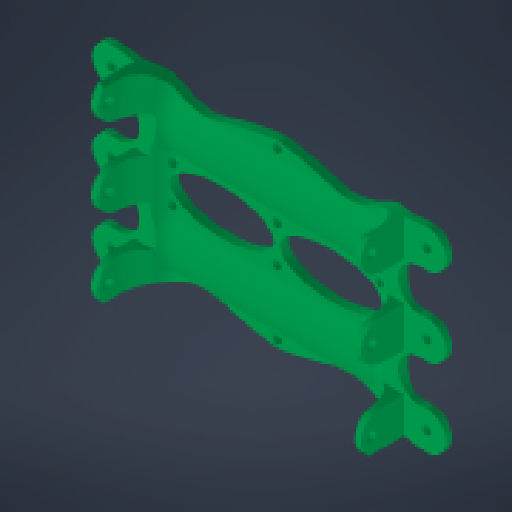
# Autodesk Inventor part: motor_holder_down
Saved by Autodesk Inventor 2024 (Build 280153000, 153)
## iProperties
Created: 2023-09-25
Part Number: motor_holder_down
Material: Типовые
Document SubType Name: Modeling
Designer: user
Mass: 66.3399 g
Surface Area: 381.903 cm^2
Volume: 66.3399 cm^3
Density: 1 g/cm^3
Appearance: По умолчанию
Author: user
Autodesk Inventor part; units mm, degrees
ref_plane "YZ Plane" through (0, 0, 0) normal (1, 0, 0) x (0, 1, 0)
sketch "Эскиз1" plane through (0, 0, 0) normal (0, 0, 1) x (1, 0, 0)
  line L0 (0, 0) -> (0, 20)
  line L1 (0, 20) -> (-20, 20)
  line L2 (-20, 20) -> (-20, 23)
  line L3 (-20, 23) -> (0, 23)
  line L4 (10, 27.5) -> (60, 27.5)
  line L5 (60, 27.5) -> (60, 23.5)
  line L6 (3, 23.5) -> (60, 23.5)
  line L7 (0, 23) -> (10, 27.5)
  line L8 (3, 23.5) -> (3, 0)
  line L9 (3, 0) -> (0, 0)
  dimension "d1" = 20
  dimension "d2" = 20
  dimension "d5" = 3
  dimension "d41" = 4
  dimension "d42" = 60
  dimension "d43" = 50
  dimension "d45" = 3
  dimension "d46" = 23.5
  constraints: 20 end point, 5 perpendicular, 3 horizontal, 1 vertical, 1 vertical alignment
  measures "d1" distance of L0.end L1.end
  measures "d2" distance of L0.start L0.end
  measures "d5" distance of L1.end L2.end
  measures "d41" distance of L4.end L5.end
  measures "d42" horizontal distance of L3.end L4.end
  measures "d43" distance of L4.start L4.end
  measures "d45" distance of L8.end L0.start
  measures "d46" distance of L6.start L8.end
extrude "Выдавливание1" add sketch "Эскиз1" along normal blind 90
ref_plane "РабПлоскость1" through (0, 0, 45) normal (0, 0, 1) x (1, 0, 0)
sketch "Эскиз2" plane through (60, 23.5, 0) normal (1, 0, 0) x (0, 0, -1)
  line L0 (0, 4) -> (-90, 4) construction
  arc A0 (-32.8167, 4) -> (-11.1833, 4) centre (-22, 22) ccw
  line L1 (0, 4) -> (-90, 4) construction
  arc A1 (-11.1833, 4) -> (-32.8167, 4) centre (-22, 22) ccw construction
  arc A2 (-78.8167, 4) -> (-57.1833, 4) centre (-68, 22) ccw
  arc A3 (-57.1833, 4) -> (-78.8167, 4) centre (-68, 22) ccw construction
  line L2 (-68, 22) -> (-22, 22) construction
  line L3 (-11.1833, 4) -> (-32.8167, 4)
  line L4 (-57.1833, 4) -> (-78.8167, 4)
  point P0 (0, -23.5)
  point P1 (-45, 22)
  point P2 (-45, 4)
  point P3 (-57.1833, 4)
  dimension "d38" = 21
  dimension "d39" = 46
  dimension "d40" = 18
  constraints: 9 point on circle, 7 point on line, 6 end point, 4 centre point, 2 coincident, 2 concentric, 2 midpoint, 1 collinear, 1 equal radius, 1 horizontal, 1 horizontal alignment, 1 vertical alignment
  measures "d38" radius of A1
  measures "d39" distance of A0.centre A2.centre
  measures "d40" vertical distance of L0.end A2.centre
extrude "Выдавливание3" cut sketch "Эскиз2" against normal through all
sketch "Эскиз10" plane through (3, 0, 90) normal (1, 0, 0) x (0, 0, -1)
  circle A0 centre (10, 5.75) radius 2
  circle A1 centre (45, 5.75) radius 2
  circle A2 centre (80, 5.75) radius 2
  line L0 (0, 0) -> (0, 23.5) projected
  line L1 (10, 5.75) -> (45, 5.75) construction
  line L2 (45, 5.75) -> (80, 5.75) construction
  point P0 (90, 0)
  point P1 (0, 5.75)
  point P2 (0, 11.5)
  dimension "d48" = 4
  dimension "d49" = 10
  dimension "d50" = 10
  constraints: 4 end point, 3 centre point, 2 collinear, 2 equal radius, 2 horizontal alignment, 1 horizontal, 1 point on line
  measures "d48" diameter of A0
  measures "d49" horizontal distance of L0.start L1.start
  measures "d50" horizontal distance of point (90, 0) L2.end
extrude "Выдавливание8" cut sketch "Эскиз10" against normal through all
sketch "Эскиз11" plane through (-20, 23, 0) normal (0, 1, 0) x (1, 0, 0)
  circle A0 centre (10, -80) radius 2
  circle A1 centre (10, -45) radius 2
  circle A2 centre (10, -10) radius 2
  line L0 (20, -90) -> (0, -90) projected
  line L1 (20, 0) -> (0, 0) projected
  line L2 (10, -80) -> (10, -45) construction
  line L3 (10, -10) -> (10, -45) construction
  point P0 (10, -90)
  dimension "d53" = 10
  dimension "d54" = 10
  dimension "d55" = 4
  constraints: 4 end point, 3 centre point, 3 vertical alignment, 2 collinear, 2 equal radius, 1 midpoint, 1 vertical
  measures "d53" horizontal distance of L0.end L2.start
  measures "d54" distance from line of L1 L3.start
  measures "d55" diameter of A2
extrude "Выдавливание9" cut sketch "Эскиз11" against normal through all
fillet "Сопряжение2" radius 15 1 edges at (0, 23, 45)
sketch "Эскиз12" plane through (60, 23.5, 0) normal (1, 0, 0) x (0, 0, -1)
  line L0 (0, 0) -> (-90, 0) projected
  arc A0 (-78.8167, 0) -> (-57.1833, 0) centre (-68, 27.9821) ccw
  arc A1 (-32.8167, 0) -> (-11.1833, 0) centre (-22, 27.9821) ccw
  point P0 (-11.1833, 4)
  point P1 (-32.8167, 4)
  point P2 (-57.1833, 4)
  point P3 (-78.8167, 4)
  dimension "d60" = 30
  dimension "d61" = 30
  constraints: 4 point on circle, 4 point on line, 4 vertical alignment, 2 centre point
  measures "d60" radius of A0
  measures "d61" radius of A1
extrude "Выдавливание10" add sketch "Эскиз12" against normal up to surface (57 mm away)
fillet "Сопряжение3" radius 13 5 edges at (3, 21.4821, 68) (3, 21.4821, 22) (3, 23.5, 45) (3, 23.5, 5.5917) (3, 23.5, 84.4083)
mirror "Зеркальное отражение9" about plane through (60, 23.5, 0) normal (1, 0, 0) of "Выдавливание3", "Выдавливание8", "Выдавливание9", "Сопряжение2", "Выдавливание10", "Сопряжение3", "Выдавливание1"
sketch "Эскиз13" plane through (120, 0, 0) normal (1, 0, 0) x (0, 0, -1)
  line L0 (0, 20) -> (-90, 20) projected
  line L1 (0, 20) -> (-90, 20) projected
  line L2 (-54, 20) -> (-54, 10)
  line L3 (-36, 20) -> (-36, 10)
  arc A0 (-54, 10) -> (-36, 10) centre (-45, 10) ccw
  line L4 (-71, 20) -> (-71, 10)
  line L5 (-89, 20) -> (-89, 10)
  line L6 (-19, 20) -> (-19, 10)
  line L7 (-1, 20) -> (-1, 10)
  arc A1 (-89, 10) -> (-71, 10) centre (-80, 10) ccw
  arc A2 (-19, 10) -> (-1, 10) centre (-10, 10) ccw
  circle A3 centre (-80, 5.75) radius 2 projected
  circle A4 centre (-10, 5.75) radius 2 projected
  line L8 (-90, 20) -> (-90, 0) projected
  line L9 (0, 0) -> (-90, 0) projected
  line L10 (0, 20) -> (0, 0) projected
  point P0 (-45, 20)
  point P1 (-45, 20)
  dimension "d65" = 18
  dimension "d67" = 18
  dimension "d68" = 18
  dimension "d69" = 10
  constraints: 12 end point, 6 point on circle, 6 tangent, 5 vertical, 3 centre point, 3 vertical alignment, 1 horizontal alignment, 1 parallel, 1 perpendicular, 9 other
  measures "d65" distance between parallel lines of L3 L2
  measures "d67" distance between parallel lines of L5 L4
  measures "d68" distance of L7.start L6.start
  measures "d69" distance of L2.start L2.end
extrude "Выдавливание11" cut sketch "Эскиз13" against normal through all contours L10 L9 L8 L0 L5 A1 L4 L2 A0 L3 L6 A2 L7
sketch "Эскиз15" plane through (10, 27.5, 11.1833) normal (0, 1, 0) x (1, 0, 0)
  circle A0 centre (-20, 1.1833) radius 2 projected
  circle A1 centre (-20, -33.8167) radius 2 projected
  circle A2 centre (-20, -68.8167) radius 2 projected
  arc A3 (-19.2944, 9.654) -> (-18.446, -7.1734) centre (-20, 1.1833) ccw
  arc A4 (-18.446, -25.4599) -> (-18.446, -42.1734) centre (-20, -33.8167) ccw
  arc A5 (-18.446, -60.4599) -> (-19.2944, -77.2873) centre (-20, -68.8167) ccw
  arc A6 (-18.446, -25.4599) -> (-18.446, -7.1734) centre (-16.7458, -16.3167) ccw
  arc A7 (-18.446, -60.4599) -> (-18.446, -42.1734) centre (-16.7458, -51.3167) ccw
  line L0 (100, -67.6333) -> (0, -67.6333) projected
  line L1 (-30, 11.1833) -> (-30, -78.8167) projected
  line L2 (6, 11.1833) -> (94, 11.1833) projected
  line L3 (0, -78.8167) -> (100, -78.8167) projected
  line L4 (0, 11.1833) -> (100, 11.1833) projected
  line L5 (0, 11.1833) -> (-7.0641, 11.1833) projected
  line L6 (-7.0641, 11.1833) -> (-13.2195, 11.1833) projected
  line L7 (-13.2195, 11.1833) -> (-30, 11.1833) projected
  line L8 (-13.2195, -78.8167) -> (-30, -78.8167) projected
  line L9 (-13.2195, -78.8167) -> (-7.0641, -78.8167) projected
  line L10 (0, -78.8167) -> (-7.0641, -78.8167) projected
  arc A8 (7, 2.1833) -> (-19.2944, 9.654) centre (-25.1885, -61.1009) ccw
  arc A9 (-19.2944, -77.2873) -> (7, -69.8167) centre (-25.1885, -6.5324) ccw
  line L11 (7, 2.1833) -> (7, 11.1833)
  line L12 (7, -69.8167) -> (7, -78.8167)
  point P0 (-10, 11.1833)
  point P1 (-30, -33.8167)
  dimension "d72" = 17
  dimension "d73" = 9.3
  dimension "d79" = 9
  dimension "d80" = 37
  dimension "d81" = 71
  constraints: 14 point on circle, 7 centre point, 6 tangent, 4 end point, 3 coincident, 3 equal radius, 2 perpendicular, 2 point on line, 2 vertical alignment, 1 collinear, 1 midpoint
  measures "d72" diameter of A3
  measures "d73" radius of A7
  measures "d79" distance of L11.start L11.end
  measures "d80" distance of L1.start L11.end
  measures "d81" radius of A9
extrude "Выдавливание12" cut sketch "Эскиз15" against normal through all contours A3 A6 A4 A7 A5 A9 L12 L3 L10 L9 L8 L1 L7 L6 L5 L4 L2 L11 A8
ref_plane "РабПлоскость3" through (60, 10, 54) normal (-1, 0, 0) x (0, 0, 1)
mirror "Зеркальное отражение10" about plane through (60, 10, 54) normal (-1, 0, 0) of "Выдавливание12"
sketch "Эскиз16" plane through (10, 27.5, 57.1833) normal (0, 1, 0) x (1, 0, 0)
  arc A0 (7, 48.1833) -> (0, 51.2808) centre (-25.1885, -15.1009) ccw projected
  arc A1 (7, 48.1833) -> (26.0438, 46.6851) centre (18.334, 70.4665) ccw
  arc A2 (50, 52.1833) -> (26.0438, 46.6851) centre (69.2187, -86.4912) ccw
  line L0 (7, 57.1833) -> (93, 57.1833) projected
  line L1 (50, 52.1833) -> (50, 57.1833)
  line L2 (7, 57.1833) -> (7, 48.1833) projected
  point P0 (-10, 57.1833)
  dimension "d82" = 25
  dimension "d83" = 140
  dimension "d84" = 5
  constraints: 4 point on circle, 2 centre point, 2 end point, 2 tangent, 1 midpoint, 1 vertical, 1 vertical alignment
  measures "d82" radius of A1
  measures "d83" radius of A2
  measures "d84" distance of L1.start L1.end
extrude "Выдавливание13" cut sketch "Эскиз16" against normal through all
mirror "Зеркальное отражение11" about plane through (60, 10, 54) normal (-1, 0, 0) of "Выдавливание13"
mirror "Зеркальное отражение12" about plane through (0, 0, 45) normal (0, 0, 1) of "Выдавливание13", "Зеркальное отражение11"
sketch "Эскиз17" plane through (10, 27.5, 57.1833) normal (0, 1, 0) x (1, 0, 0)
  ellipse E0 centre (25.7195, 12.1833) end of major axis (48.7195, 12.1833) minor radius 10
  line L0 (113.2195, 3.2889) -> (113.2195, 21.0778) projected
  point P0 (-10, 57.1833)
  point P1 (113.2195, 12.1833)
  dimension "d88" = 23
  dimension "d89" = 10
  dimension "d90" = 87.5
  constraints: 1 centre point, 1 horizontal alignment, 1 midpoint, 1 other
  measures "d89" radius of E0
  measures "d90" distance of point (113.22, 12.183) E0.centre
extrude "Выдавливание14" cut sketch "Эскиз17" against normal through all
mirror "Зеркальное отражение13" about plane through (60, 10, 54) normal (-1, 0, 0) of "Выдавливание14"
fillet "Сопряжение4" radius 15 2 edges at (60, 25.5, 85) (60, 25.5, 5)
sketch "Эскиз18" plane through (33.471, 27.5, 78.8167) normal (0, 1, 0) x (1, 0, 0)
  circle A0 centre (26.529, 42) radius 2
  circle A1 centre (-19.471, 42) radius 2
  circle A2 centre (72.529, 42) radius 2
  circle A3 centre (26.529, 70.6558) radius 2
  arc A4 (28.8353, 73.4774) -> (24.2228, 73.4774) centre (26.529, 58.6558) ccw projected
  line L0 (76.529, 46) -> (-23.471, 46) projected
  line L1 (-23.471, 46) -> (-23.471, 21.6333) projected
  line L2 (76.529, 46) -> (76.529, 21.6333) projected
  point P0 (-33.471, 78.8167)
  point P1 (26.529, 73.6558)
  point P2 (26.529, 73.6558)
  dimension "d95" = 4
  dimension "d96" = 4
  dimension "d97" = 4
  dimension "d98" = 4
  dimension "d99" = 3
  constraints: 4 centre point, 3 equal radius, 2 horizontal alignment, 2 point on circle, 2 vertical alignment
  measures "d95" diameter of A3
  measures "d96" distance from line of L0 A1.centre
  measures "d97" distance from line of L1 A1.centre
  measures "d98" distance from line of L2 A2.centre
  measures "d99" distance of point (26.529, 73.656) A3.centre
extrude "Выдавливание15" cut sketch "Эскиз18" against normal through all
mirror "Зеркальное отражение14" about plane through (0, 0, 45) normal (0, 0, 1) of "Выдавливание15"
sketch "Эскиз19" plane through (120, 10, 71) normal (1, 0, 0) x (0, 0, -1)
  line L0 (68.0721, 10) -> (52, 10) projected
  line L1 (68.0721, 10) -> (52, 10)
  line L2 (52, 10) -> (52, -9)
  line L3 (52, -9) -> (68.0721, -9)
  line L4 (68.0721, -9) -> (68.0721, 10)
  line L5 (52, 10) -> (52, 0) projected
  arc A0 (52, 0) -> (68.0721, -5.5664) centre (61, 0) ccw projected
  constraints: 8 end point, 2 parallel, 1 horizontal, 1 perpendicular, 1 point on line, 1 tangent
extrude "Выдавливание16" cut sketch "Эскиз19" against normal through all
mirror "Зеркальное отражение15" about plane through (0, 0, 45) normal (0, 0, 1) of "Выдавливание16"
